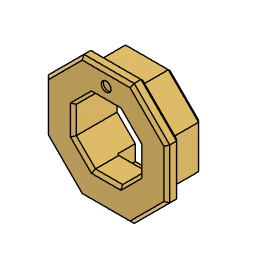
Multiboard - Toothbrush v5 (Autodesk Fusion 360 archive; units mm, degrees)
design "Multiboard - Adapter"
Autodesk Fusion 360 part; units mm, degrees
sketch "Base" plane through (0, 0, 0) normal (0, 1, 0) x (1, 0, 0) in component "Squeegee Holder"
  line L0 (4.4321, 10.7) -> (-4.4321, 10.7)
  line L1 (-4.4321, 10.7) -> (-10.7, 4.4321)
  line L2 (-10.7, 4.4321) -> (-10.7, -4.4321)
  line L3 (-10.7, -4.4321) -> (-4.4321, -10.7)
  line L4 (-4.4321, -10.7) -> (4.4321, -10.7)
  line L5 (4.4321, -10.7) -> (10.7, -4.4321)
  line L6 (10.7, -4.4321) -> (10.7, 4.4321)
  line L7 (10.7, 4.4321) -> (4.4321, 10.7)
  line L8 (10.65, 4.4114) -> (4.4114, 10.65)
  line L9 (4.4114, 10.65) -> (-4.4114, 10.65)
  line L10 (-4.4114, 10.65) -> (-10.65, 4.4114)
  line L11 (-10.65, 4.4114) -> (-10.65, -4.4114)
  line L12 (-10.65, -4.4114) -> (-4.4114, -10.65)
  line L13 (-4.4114, -10.65) -> (4.4114, -10.65)
  line L14 (4.4114, -10.65) -> (10.65, -4.4114)
  line L15 (10.65, -4.4114) -> (10.65, 4.4114)
  line L16 (12.5, 5.1777) -> (5.1777, 12.5)
  line L17 (5.1777, 12.5) -> (-5.1777, 12.5)
  line L18 (-5.1777, 12.5) -> (-12.5, 5.1777)
  line L19 (-12.5, 5.1777) -> (-12.5, -5.1777)
  line L20 (-12.5, -5.1777) -> (-5.1777, -12.5)
  line L21 (-5.1777, -12.5) -> (5.1777, -12.5)
  line L22 (5.1777, -12.5) -> (12.5, -5.1777)
  line L23 (12.5, -5.1777) -> (12.5, 5.1777)
  line L24 (6.75, 2.7959) -> (2.7959, 6.75)
  line L25 (2.7959, 6.75) -> (-2.7959, 6.75)
  line L26 (-2.7959, 6.75) -> (-6.75, 2.7959)
  line L27 (-6.75, 2.7959) -> (-6.75, -2.7959)
  line L28 (-6.75, -2.7959) -> (-2.7959, -6.75)
  line L29 (-2.7959, -6.75) -> (2.7959, -6.75)
  line L30 (2.7959, -6.75) -> (6.75, -2.7959)
  line L31 (6.75, -2.7959) -> (6.75, 2.7959)
  line L32 (-4.9706, 12) -> (-12, 4.9706)
  line L33 (-12, 4.9706) -> (-12, -4.9706)
  line L34 (-12, -4.9706) -> (-4.9706, -12)
  line L35 (-4.9706, -12) -> (4.9706, -12)
  line L36 (4.9706, -12) -> (12, -4.9706)
  line L37 (12, -4.9706) -> (12, 4.9706)
  line L38 (12, 4.9706) -> (4.9706, 12)
  line L39 (4.9706, 12) -> (-4.9706, 12)
  dimension "d4" = 21.4
  dimension "d5" = 25
  dimension "d56" = 13.5
  dimension "d66" = 24
  constraint horizontal L0
  constraint horizontal L17
  constraint horizontal L25
  constraint horizontal L39
  measures "d4" distance of L2 L6
  measures "d5" distance of L19 L23
  measures "d56" distance of L27 L31
  measures "d66" distance of L33 L37
sketch "Notch" plane through (0, 0, 0) normal (0, 1, 0) x (1, 0, 0) in component "Squeegee Holder"
  line L0 (-4.4114, -10.65) -> (4.4114, -10.65) construction
  line L1 (3, -6.75) -> (-3, -6.75) construction
  line L2 (-3, -6.75) -> (-3, -9.75)
  line L3 (-3, -9.75) -> (3, -9.75)
  line L4 (3, -9.75) -> (3, -6.75)
  line L5 (-3, -6.75) -> (-3, -6.25)
  line L6 (3, -6.75) -> (3, -6.25)
  line L7 (3, -6.25) -> (-3, -6.25)
  line L8 (3, 9.75) -> (-3, 9.75)
  line L9 (-3, 9.75) -> (-3, 6.75)
  line L10 (3, 6.75) -> (3, 9.75)
  line L11 (3, 6.75) -> (3, 6.25)
  line L12 (-3, 6.75) -> (-3, 6.25)
  line L13 (-3, 6.25) -> (3, 6.25)
  line L14 (-2.7959, -6.75) -> (2.7959, -6.75)
  dimension "d24" = 6
  dimension "d25" = 3
  dimension "d31" = 360
  dimension "d57" = 0.5
  constraint horizontal L1
  constraint vertical L2
  constraint horizontal L3
  constraint vertical L4
  constraint midpoint L1 L14
  constraint perpendicular L1 L5
  constraint perpendicular L1 L6
  constraint horizontal L7
  measures "d24" distance of L1.start L1.end
  measures "d25" distance of L1 L3
  measures "d57" distance of L1.start L6.end
extrude "Extrude5" add sketch "Base" along normal blind 6.4 contours L8 L9 L10 L11 L12 L13 L14 L15 | L24 L25 L26 L27 L28 L29 L30 L31 in component "Squeegee Holder"
extrude "Extrude10" add sketch "Base" against normal blind 2.6 contours L0 L1 L2 L3 L4 L5 L6 L7 | L8 L9 L10 L11 L12 L13 L14 L15 | L16 L17 L18 L19 L20 L21 L22 L23 | L24 L25 L26 L27 L28 L29 L30 L31 | L32 L33 L34 L35 L36 L37 L38 L39 in component "Squeegee Holder"
extrude "Extrude6" cut sketch "Base" along normal through all and the other way through all contours L24 L25 L26 L27 L28 L29 L30 L31 in component "Squeegee Holder"
extrude "Extrude8" cut sketch "Notch" against normal blind 3.6 from surface at 6.4 in component "Squeegee Holder"
sketch "Marca" plane through (0, -2.6, 0) normal (0, 1, 0) x (1, 0, 0) in component "Squeegee Holder"
  circle A0 centre (0, -9.625) radius 1
  line L0 (-2.7959, 6.75) -> (-6.75, 2.7959)
  line L1 (-6.75, 2.7959) -> (-6.75, -2.7959)
  line L2 (-6.75, -2.7959) -> (-2.7959, -6.75)
  line L3 (-2.7959, -6.75) -> (2.7959, -6.75)
  line L4 (2.7959, -6.75) -> (6.75, -2.7959)
  line L5 (6.75, -2.7959) -> (6.75, 2.7959)
  line L6 (6.75, 2.7959) -> (2.7959, 6.75)
  line L7 (2.7959, 6.75) -> (-2.7959, 6.75)
  line L8 (12.5, 5.1777) -> (12.5, -5.1777)
  line L9 (12.5, -5.1777) -> (5.1777, -12.5)
  line L10 (5.1777, -12.5) -> (-5.1777, -12.5)
  line L11 (-5.1777, -12.5) -> (-12.5, -5.1777)
  line L12 (-12.5, -5.1777) -> (-12.5, 5.1777)
  line L13 (-12.5, 5.1777) -> (-5.1777, 12.5)
  line L14 (-5.1777, 12.5) -> (5.1777, 12.5)
  line L15 (5.1777, 12.5) -> (12.5, 5.1777)
  line L16 (0, -12.5) -> (0, -6.75) construction
  dimension "d61" = 2
  constraint midpoint L10 L16.start
  constraint midpoint L3 L16.end
  constraint midpoint A0.centre L16
  measures "d61" diameter of A0
extrude "Extrude9" cut sketch "Marca" along normal blind 0.4 contours A0 in component "Squeegee Holder"
chamfer "Chamfer3" distance 0.6 angle 45 32 edges at (0, 6.4, 10.65) (7.5307, 6.4, 7.5307) (10.65, 6.4, 0) (7.5307, 6.4, -7.5307) (0, 6.4, -10.65) (-7.5307, 6.4, -7.5307) (-10.65, 6.4, 0) (-7.5307, 6.4, 7.5307) (12.5, 0, 0) (8.8388, 0, 8.8388) (8.8388, -2.6, 8.8388) (12.5, -2.6, 0) (0, 0, 12.5) (0, -2.6, 12.5) (8.8388, 0, -8.8388) (8.8388, -2.6, -8.8388) (0, -2.6, -12.5) (0, 0, -12.5) (-8.8388, 0, -8.8388) (-8.8388, -2.6, -8.8388) (-12.5, -2.6, 0) (-12.5, 0, 0) (-8.8388, 0, 8.8388) (-8.8388, -2.6, 8.8388) (0, -2.6, 6.75) (4.773, -2.6, 4.773) (6.75, -2.6, 0) (4.773, -2.6, -4.773) (0, -2.6, -6.75) (-4.773, -2.6, -4.773) (-6.75, -2.6, 0) (-4.773, -2.6, 4.773) in component "Squeegee Holder"
component "Squeegee Holder" placed x (1, 0, 0) y (0, 1, 0) z (0, 0, 1) at (0, 0, 0)
equation "d2 = -Clearance_Tight"
equation "d31 = 360.00 °"
equation "Clearance_Tight = 0.05 mm"
named bodies: "Multiboard - Adapter"
